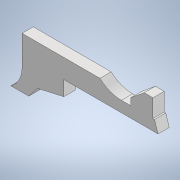
# Autodesk Inventor part: inner slider
Saved by Autodesk Inventor 2022 (Build 260153000, 153)
## iProperties
Created: 2022-05-17
Part Number: inner slider
Material: Generic
Document SubType Name: Sheet Metal
Designer: joshn
Density: 1 g/cm^3
Sheet Metal Rule: Default
Appearance: Default
Author: joshn
Autodesk Inventor part; units mm, degrees
ref_plane "YZ Plane" through (0, 0, 0) normal (1, 0, 0) x (0, 1, 0)
ref_plane "XZ Plane" through (0, 0, 0) normal (0, 1, 0) x (-1, 0, 0)
ref_plane "XY Plane" through (0, 0, 0) normal (0, 0, 1) x (1, 0, 0)
sketch "Sketch1" plane through (0, 0, 0) normal (0, 0, 1) x (1, 0, 0)
  line L0 (-27.669, 21.4051) -> (50.2215, 21.4051) construction
  line L1 (50.2215, 21.4051) -> (50.2215, -35.1456) construction
  line L2 (50.2215, -35.1456) -> (-27.669, -35.1456) construction
  line L3 (-27.669, -35.1456) -> (-27.669, 21.4051) construction
  line L4 (-25.2081, -35.2295) -> (52.6824, -35.2295) construction
  line L5 (16.9988, 9.3626) -> (27.4291, 9.3626)
  line L6 (30.2909, 8.2443) -> (31.5557, 8.2443)
  line L7 (31.5557, 8.2443) -> (31.5557, 9.1701)
  line L8 (31.5557, 9.1701) -> (33.3477, 10.6493)
  line L9 (33.3477, 10.6493) -> (34.52, 10.6493)
  line L10 (34.52, 10.6493) -> (34.52, 8.2443)
  line L11 (34.52, 8.2443) -> (34.7306, 8.2443)
  line L12 (34.7306, 8.2443) -> (35.1991, 6.7921)
  line L13 (35.1991, 6.7921) -> (22.5878, 6.7921)
  line L14 (22.5878, 6.7921) -> (22.5878, 4.8059)
  line L15 (22.5878, 4.8059) -> (19.0643, 4.0103)
  line L16 (19.0643, 4.0103) -> (17.8875, 2.5188)
  line L17 (17.8875, 2.5188) -> (15.4819, 2.5188)
  line L18 (16.9988, 9.3626) -> (16.9988, 5.4381)
  arc A0 (15.4819, 2.5188) -> (16.9988, 5.4381) centre (13.4312, 5.4381) ccw
  arc A1 (27.4291, 9.3626) -> (30.2909, 8.2443) centre (30.2909, 12.4655) ccw
  line L19 (36.8494, 6.7921) -> (35.3044, 6.7921)
  line L20 (36.8494, 6.7921) -> (35.3044, 6.7921) construction
  line L21 (36.8494, 6.7921) -> (35.3044, 6.7921) construction
  point P0 (0, 0)
  point P1 (26.4448, 6.7921)
  dimension "d1" = 77.8905
  dimension "d2" = 77.8905
  measures "d1" distance of L4.start L4.end
  measures "d2" distance of L1.end L2.end
extrude "Plate1" add sketch "Sketch1" along normal blind 1.5
equation "\"d2\" = d1"
equation "\"d31\" = Thickness"
equation "\"BendRadius\" = Thickness"
equation "\"BendReliefWidth\" = Thickness"
equation "\"BendReliefDepth\" = 0.5 * Thickness"
equation "\"CornerReliefSize\" = 4 * Thickness"
equation "\"MinimumRemnant\" = 2 * Thickness"
equation "\"TransitionRadius\" = BendRadius"
equation "\"JacobiRadiusSize\" = BendRadius"
equation "\"GapSize\" = Thickness"
equation "\"Thickness\" = 1.5"
body "Solid1"
